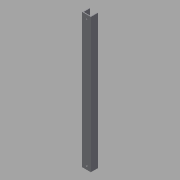
# Autodesk Inventor part: 19in c-channel
Saved by Autodesk Inventor 2013 (Build 170138000, 138)
## iProperties
Created: 2013-01-08
Part Number: 19in c-channel
Material: Generic
Document SubType Name: Modeling
Designer: Naphat
Density: 1 g/cm^3
Author: Naphat
Autodesk Inventor part; units mm, degrees
ref_plane "YZ Plane" through (0, 0, 0) normal (1, 0, 0) x (0, 1, 0)
ref_plane "XZ Plane" through (0, 0, 0) normal (0, 1, 0) x (-1, 0, 0)
ref_plane "XY Plane" through (0, 0, 0) normal (0, 0, 1) x (1, 0, 0)
sketch "Sketch1" plane through (0, 0, 0) normal (0, 0, 1) x (1, 0, 0)
  line L0 (-15.7, 12.7) -> (-12.7, 12.7)
  line L1 (-12.7, 12.7) -> (-12.7, -9.7)
  line L2 (-12.7, -9.7) -> (12.7, -9.7)
  line L3 (12.7, -9.7) -> (12.7, 12.7)
  line L4 (12.7, 12.7) -> (15.7, 12.7)
  line L5 (15.7, 12.7) -> (15.7, -12.7)
  line L6 (15.7, -12.7) -> (-15.7, -12.7)
  line L7 (-15.7, -12.7) -> (-15.7, 12.7)
  point P0 (0, 0)
  dimension "d0" = 3
  dimension "d2" = 3
  dimension "d3" = 25.4
  dimension "d4" = 31.4
  dimension "d5" = 15.7
  dimension "d7" = 12.7
  dimension "d8" = 3
  constraints: 16 end point, 5 parallel, 1 collinear, 1 horizontal, 1 perpendicular
  measures "d0" distance of L0.start L0.end
  measures "d2" distance of L3.end L4.end
  measures "d3" distance of L6.end L0.start
  measures "d4" distance of L5.end L6.end
  measures "d5" distance from line of point (0, 0) L7
  measures "d7" distance from line of L6 point (0, 0)
  measures "d8" distance between parallel lines of L6 L2
extrude "Extrusion1" add sketch "Sketch1" against normal blind 482.6
sketch "Sketch3" plane through (-12.7, -9.7, 0) normal (0, 1, 0) x (1, 0, 0)
  line L0 (0, 0) -> (25.4, 0) projected
  line L1 (25.4, 0) -> (25.4, 482.6) projected
  line L2 (0, 482.6) -> (25.4, 482.6) projected
  line L3 (0, 0) -> (0, 482.6) projected
  line L4 (0, 0) -> (0, 25.4) construction
  line L5 (0, 25.4) -> (25.4, 25.4) construction
  line L6 (25.4, 25.4) -> (25.4, 0) construction
  line L7 (25.4, 0) -> (0, 0) construction
  line L8 (12.7, 0) -> (12.7, 25.4) construction
  line L9 (0, 12.7) -> (25.4, 12.7) construction
  line L10 (0, 482.6) -> (25.4, 482.6) construction
  line L11 (25.4, 482.6) -> (25.4, 457.2) construction
  line L12 (25.4, 457.2) -> (0, 457.2) construction
  line L13 (0, 457.2) -> (0, 482.6) construction
  line L14 (12.7, 457.2) -> (12.7, 482.6) construction
  line L15 (0, 469.9) -> (25.4, 469.9) construction
  circle A0 centre (12.7, 469.9) radius 3.175
  circle A1 centre (12.7, 12.7) radius 3.175
  dimension "d15" = 25.4
  dimension "d16" = 25.4
  dimension "d17" = 6.35
  dimension "d18" = 6.35
  constraints: 24 end point, 9 midpoint, 5 perpendicular, 4 point on line, 2 centre point, 1 parallel
  measures "d15" distance of L0.start L4.end
  measures "d16" distance of L1.end L11.end
  measures "d17" diameter of A0
  measures "d18" diameter of A1
extrude "Extrusion3" cut sketch "Sketch3" against normal blind 10 contours A0 | A1
equation "\"d2\" = d0"
equation "\"d5\" = 0.5 * d4"
equation "\"d7\" = 0.5 * d3"
equation "\"d8\" = d0"
body "Solid1"
